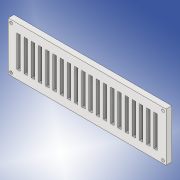
# Autodesk Inventor part: HA006
Saved by Autodesk Inventor 2017 (Build 210142000, 142)
## iProperties
Created: 2017-06-25
Part Number: HA006
Material: ABS Plastic
Document SubType Name: Modeling
Designer: Zach
Density: 1.06 g/cm^3
Appearance: CR White
Author: Zach
Autodesk Inventor part; units mm, degrees
ref_plane "YZ Plane" through (0, 0, 0) normal (1, 0, 0) x (0, 1, 0)
ref_plane "XZ Plane" through (0, 0, 0) normal (0, 1, 0) x (-1, 0, 0)
ref_plane "XY Plane" through (0, 0, 0) normal (0, 0, 1) x (1, 0, 0)
sketch "Sketch1" plane through (0, 0, 0) normal (0, 0, 1) x (1, 0, 0)
  line L0 (0, 0) -> (275, 0)
  line L1 (275, 0) -> (275, 85)
  line L2 (275, 85) -> (0, 85)
  line L3 (0, 85) -> (0, 0)
  dimension "d0" = 275
  dimension "d1" = 85
  constraints: 8 end point, 2 parallel, 1 horizontal, 1 perpendicular
  measures "d0" distance of L2.end L1.end
  measures "d1" distance of L1.end L0.end
extrude "Extrusion1" add sketch "Sketch1" along normal blind 10
sketch "Sketch2" plane through (0, 0, 10) normal (0, 0, 1) x (1, 0, 0)
  line L0 (0, 0) -> (275, 0) construction
  line L1 (275, 0) -> (275, 85) construction
  line L2 (275, 85) -> (0, 85) construction
  line L3 (0, 85) -> (0, 0) construction
  line L4 (5, 80) -> (270, 80) construction
  line L5 (270, 80) -> (270, 5) construction
  line L6 (270, 5) -> (5, 5) construction
  line L7 (5, 5) -> (5, 80) construction
  line L8 (10, 75) -> (265, 75) construction
  line L9 (265, 75) -> (265, 10) construction
  line L10 (265, 10) -> (10, 10) construction
  line L11 (10, 10) -> (10, 75) construction
  circle A0 centre (5, 80) radius 2.5
  circle A1 centre (270, 80) radius 2.5
  circle A2 centre (270, 5) radius 2.5
  circle A3 centre (5, 5) radius 2.5
  line L12 (15, 70) -> (21, 70)
  line L13 (21, 70) -> (21, 15)
  line L14 (21, 15) -> (15, 15)
  line L15 (15, 15) -> (15, 70)
  line L16 (15, 70) -> (260, 70) construction
  line L17 (260, 70) -> (260, 15) construction
  line L18 (260, 15) -> (15, 15) construction
  line L19 (15, 15) -> (15, 70) construction
  line L20 (33.57, 70) -> (33.57, 15)
  line L21 (27.57, 70) -> (33.57, 70)
  line L22 (27.57, 15) -> (27.57, 70)
  line L23 (27.57, 15) -> (27.57, 70) construction
  line L24 (33.57, 15) -> (27.57, 15)
  line L25 (46.14, 70) -> (46.14, 15)
  line L26 (40.14, 70) -> (46.14, 70)
  line L27 (40.14, 15) -> (40.14, 70)
  line L28 (40.14, 15) -> (40.14, 70) construction
  line L29 (46.14, 15) -> (40.14, 15)
  line L30 (58.71, 70) -> (58.71, 15)
  line L31 (52.71, 70) -> (58.71, 70)
  line L32 (52.71, 15) -> (52.71, 70)
  line L33 (52.71, 15) -> (52.71, 70) construction
  line L34 (58.71, 15) -> (52.71, 15)
  line L35 (71.28, 70) -> (71.28, 15)
  line L36 (65.28, 70) -> (71.28, 70)
  line L37 (65.28, 15) -> (65.28, 70)
  line L38 (65.28, 15) -> (65.28, 70) construction
  line L39 (71.28, 15) -> (65.28, 15)
  line L40 (83.85, 70) -> (83.85, 15)
  line L41 (77.85, 70) -> (83.85, 70)
  line L42 (77.85, 15) -> (77.85, 70)
  line L43 (77.85, 15) -> (77.85, 70) construction
  line L44 (83.85, 15) -> (77.85, 15)
  line L45 (96.42, 70) -> (96.42, 15)
  line L46 (90.42, 70) -> (96.42, 70)
  line L47 (90.42, 15) -> (90.42, 70)
  line L48 (90.42, 15) -> (90.42, 70) construction
  line L49 (96.42, 15) -> (90.42, 15)
  line L50 (108.99, 70) -> (108.99, 15)
  line L51 (102.99, 70) -> (108.99, 70)
  line L52 (102.99, 15) -> (102.99, 70)
  line L53 (102.99, 15) -> (102.99, 70) construction
  line L54 (108.99, 15) -> (102.99, 15)
  line L55 (121.56, 70) -> (121.56, 15)
  line L56 (115.56, 70) -> (121.56, 70)
  line L57 (115.56, 15) -> (115.56, 70)
  line L58 (115.56, 15) -> (115.56, 70) construction
  line L59 (121.56, 15) -> (115.56, 15)
  line L60 (134.13, 70) -> (134.13, 15)
  line L61 (128.13, 70) -> (134.13, 70)
  line L62 (128.13, 15) -> (128.13, 70)
  line L63 (128.13, 15) -> (128.13, 70) construction
  line L64 (134.13, 15) -> (128.13, 15)
  line L65 (146.7, 70) -> (146.7, 15)
  line L66 (140.7, 70) -> (146.7, 70)
  line L67 (140.7, 15) -> (140.7, 70)
  line L68 (140.7, 15) -> (140.7, 70) construction
  line L69 (146.7, 15) -> (140.7, 15)
  line L70 (159.27, 70) -> (159.27, 15)
  line L71 (153.27, 70) -> (159.27, 70)
  line L72 (153.27, 15) -> (153.27, 70)
  line L73 (153.27, 15) -> (153.27, 70) construction
  line L74 (159.27, 15) -> (153.27, 15)
  line L75 (171.84, 70) -> (171.84, 15)
  line L76 (165.84, 70) -> (171.84, 70)
  line L77 (165.84, 15) -> (165.84, 70)
  line L78 (165.84, 15) -> (165.84, 70) construction
  line L79 (171.84, 15) -> (165.84, 15)
  line L80 (184.41, 70) -> (184.41, 15)
  line L81 (178.41, 70) -> (184.41, 70)
  line L82 (178.41, 15) -> (178.41, 70)
  line L83 (178.41, 15) -> (178.41, 70) construction
  line L84 (184.41, 15) -> (178.41, 15)
  line L85 (196.98, 70) -> (196.98, 15)
  line L86 (190.98, 70) -> (196.98, 70)
  line L87 (190.98, 15) -> (190.98, 70)
  line L88 (190.98, 15) -> (190.98, 70) construction
  line L89 (196.98, 15) -> (190.98, 15)
  line L90 (209.55, 70) -> (209.55, 15)
  line L91 (203.55, 70) -> (209.55, 70)
  line L92 (203.55, 15) -> (203.55, 70)
  line L93 (203.55, 15) -> (203.55, 70) construction
  line L94 (209.55, 15) -> (203.55, 15)
  line L95 (222.12, 70) -> (222.12, 15)
  line L96 (216.12, 70) -> (222.12, 70)
  line L97 (216.12, 15) -> (216.12, 70)
  line L98 (216.12, 15) -> (216.12, 70) construction
  line L99 (222.12, 15) -> (216.12, 15)
  line L100 (234.69, 70) -> (234.69, 15)
  line L101 (228.69, 70) -> (234.69, 70)
  line L102 (228.69, 15) -> (228.69, 70)
  line L103 (228.69, 15) -> (228.69, 70) construction
  line L104 (234.69, 15) -> (228.69, 15)
  line L105 (247.26, 70) -> (247.26, 15)
  line L106 (241.26, 70) -> (247.26, 70)
  line L107 (241.26, 15) -> (241.26, 70)
  line L108 (241.26, 15) -> (241.26, 70) construction
  line L109 (247.26, 15) -> (241.26, 15)
  line L110 (259.83, 70) -> (259.83, 15)
  line L111 (253.83, 70) -> (259.83, 70)
  line L112 (253.83, 15) -> (253.83, 70)
  line L113 (253.83, 15) -> (253.83, 70) construction
  line L114 (259.83, 15) -> (253.83, 15)
  dimension "d4" = 5
  dimension "d5" = 10
  dimension "d6" = 5
  dimension "d7" = 5
  dimension "d8" = 5
  dimension "d9" = 5
  dimension "d10" = 6
  dimension "d11" = 15
  dimension "d14" = 12.57
  constraints: 222 end point, 4 centre point, 4 coincident, 2 horizontal, 2 parallel, 1 perpendicular, 1 point on line, 199 other
  measures "d4" distance between parallel lines of L2 L4
  measures "d5" distance between parallel lines of L2 L8
  measures "d6" diameter of A0
  measures "d7" diameter of A1
  measures "d8" diameter of A2
  measures "d9" diameter of A3
  measures "d10" distance of L14.end L13.end
  measures "d11" distance between parallel lines of L2 L16
  measures "d14" distance of L12.end L20.start
extrude "Extrusion2" cut sketch "Sketch2" against normal through all
body "Solid1"
